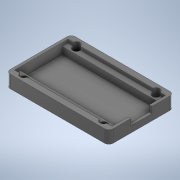
# Autodesk Inventor part: StartStopSwitch_lower_cover
Saved by Autodesk Inventor 2020.4 (Build 244396000, 396)
## iProperties
Created: 2021-10-04
Part Number: StartStopSwitch_lower_cover
Material: アセタール樹脂、黒
Document SubType Name: Modeling
Designer: Masato Kubotera
Density: 1.425 g/cm^3
Appearance: 滑らか - 黒
Description: PLA
Author: Masato Kubotera
Autodesk Inventor part; units mm, degrees
ref_plane "YZ Plane" through (0, 0, 0) normal (1, 0, 0) x (0, 1, 0)
ref_plane "XZ Plane" through (0, 0, 0) normal (0, 1, 0) x (-1, 0, 0)
ref_plane "XY Plane" through (0, 0, 0) normal (0, 0, 1) x (1, 0, 0)
derived "Switch_basis.ipt"
sketch "スケッチ1" plane through (0, 0, 0) normal (0, 0, 1) x (1, 0, 0)
  line L0 (23, 12.5) -> (23, -12.5) construction
  line L1 (23, 12.5) -> (-23, -12.5) construction
  circle A0 centre (-19, 12.5) radius 3 construction
  line L2 (-4, -9) -> (-22, -9) construction
  line L3 (-22, -9) -> (-22, 9) construction
  line L4 (-22, 9) -> (-4, 9) construction
  line L5 (-4, 9) -> (-4, -9) construction
  line L6 (-4, -9) -> (-22, 9) construction
  line L7 (-22, -9) -> (-4, 9) construction
  line L8 (-23, 0) -> (23, 0) construction
  line L9 (0, 12.5) -> (0, -12.5) construction
  line L10 (4, -9) -> (22, -9) construction
  line L11 (22, -9) -> (22, 9) construction
  line L12 (4, 9) -> (4, -9) construction
  line L13 (22, 9) -> (4, 9) construction
  line L14 (4, -9) -> (22, 9) construction
  line L15 (22, -9) -> (4, 9) construction
  line L16 (-23, 12.5) -> (23, -12.5) construction
  line L17 (-23, 12.5) -> (-20.6, 12.5) construction
  arc A1 (-20.6, 12.5) -> (-17.4, 12.5) centre (-19, 12.5) ccw construction
  arc A2 (-17.4, -12.5) -> (-20.6, -12.5) centre (-19, -12.5) ccw construction
  line L18 (-23, -12.5) -> (-20.6, -12.5) construction
  arc A3 (17.4, 12.5) -> (20.6, 12.5) centre (19, 12.5) ccw construction
  line L19 (23, 12.5) -> (20.6, 12.5) construction
  line L20 (23, -12.5) -> (20.6, -12.5) construction
  arc A4 (20.6, -12.5) -> (17.4, -12.5) centre (19, -12.5) ccw construction
  line L21 (-17.4, 12.5) -> (17.4, 12.5) construction
  line L22 (17.4, -12.5) -> (-17.4, -12.5) construction
  line L23 (-23, 12.5) -> (-23, -12.5) construction
  line L24 (-24.5, 15.5) -> (24.5, 15.5)
  line L25 (24.5, 15.5) -> (24.5, -15.5)
  line L26 (24.5, -15.5) -> (-24.5, -15.5)
  line L27 (-24.5, -15.5) -> (-24.5, 15.5)
  line L28 (-24.5, 15.5) -> (24.5, -15.5) construction
  line L29 (24.5, 15.5) -> (-24.5, -15.5) construction
  line L30 (-23.25, 12.75) -> (23.25, 12.75)
  line L31 (23.25, 12.75) -> (23.25, -12.75)
  line L32 (23.25, -12.75) -> (-23.25, -12.75)
  line L33 (-23.25, -12.75) -> (-23.25, 12.75)
  line L34 (-23.25, 12.75) -> (23.25, -12.75) construction
  line L35 (23.25, 12.75) -> (-23.25, -12.75) construction
  circle A5 centre (-19, 12.5) radius 1.75
  circle A6 centre (-19, -12.5) radius 1.75
  circle A7 centre (19, 12.5) radius 1.75
  circle A8 centre (19, -12.5) radius 1.75
  line L36 (-23.25, 10) -> (23.25, 10)
  line L37 (-23.25, -10) -> (23.25, -10)
  line L38 (23.25, 5) -> (24.5, 5)
  line L39 (23.25, -5) -> (24.5, -5)
  circle A9 centre (19, 12.5) radius 3 construction
  circle A10 centre (-19, -12.5) radius 3 construction
  circle A11 centre (19, -12.5) radius 3 construction
  point P0 (0, 0)
  point P1 (-13, 0)
  point P2 (13, 0)
  point P3 (-13, 0)
  point P4 (0, 0)
  point P5 (0, 0)
  point P6 (20.7321, -12.75)
  point P7 (17.2679, -12.75)
  point P8 (-17.2679, -12.75)
  point P9 (-20.7321, -12.75)
  point P10 (-20.7321, 12.75)
  point P11 (-17.2679, 12.75)
  point P12 (17.2679, 12.75)
  point P13 (20.7321, 12.75)
  dimension "d1" = 3.5
  dimension "d3" = 20
  dimension "d4" = 10
  measures "d1" diameter of A5
  measures "d3" distance of L36.end L37.end
  measures "d4" distance of L39.end L38.end
extrude "押し出し1" add sketch "スケッチ1" along normal blind 6 contours L24 L25 L38 L31 L30 A7 A5 L33 L32 A6 A8 L39 L26 L27
extrude "押し出し2" add sketch "スケッチ1" along normal blind 4.4 contours L36 L33 L30 A5 A7 L31 | L31 L32 A8 A6 L33 L37
extrude "押し出し3" add sketch "スケッチ1" along normal blind 1 contours L31 L37 L33 L36
fillet "フィレット1" radius 2 4 edges at (-24.5, 15.5, 3) (-24.5, -15.5, 3) (24.5, 15.5, 3) (24.5, -15.5, 3)
extrude "押し出し4" add sketch "スケッチ1" along normal blind 3 contours L25 L39 L31 L38
